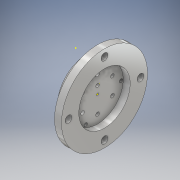
# Autodesk Inventor part: InnerSleeveFront
Saved by Autodesk Inventor 2017.3 (Build 213256000, 256)
## iProperties
Created: 2017-02-02
Part Number: InnerSleeveFront
Material: Generic
Document SubType Name: Modeling
Designer: Mac
Density: 1 g/cm^3
Appearance: Aluminum - Dark
Author: Mac
Autodesk Inventor part; units mm, degrees
ref_plane "YZ Plane" through (0, 0, 0) normal (1, 0, 0) x (0, 1, 0)
ref_plane "XZ Plane" through (0, 0, 0) normal (0, 1, 0) x (-1, 0, 0)
sketch "Sketch1" plane through (0, 0, 0) normal (1, 0, 0) x (0, 1, 0)
  circle A0 centre (0, 0) radius 13.2
  dimension "d0" = 26.4
  constraints: 1 centre point, 1 coincident
  measures "d0" diameter of A0
extrude "Extrusion1" add sketch "Sketch1" along normal blind 100
sketch "Sketch5" plane through (100, 0, 0) normal (1, 0, 0) x (0, 0, -1)
  line L0 (-14, -7) -> (14, -7)
  line L1 (14, -7) -> (14, 7)
  line L2 (14, 7) -> (-14, 7)
  line L3 (-14, 7) -> (-14, -7)
  line L4 (-7, -14) -> (7, -14)
  line L5 (7, -14) -> (7, 14)
  line L6 (7, 14) -> (-7, 14)
  line L7 (-7, 14) -> (-7, -14)
  point P0 (0, 0)
  constraints: 16 end point, 4 parallel, 2 horizontal, 2 perpendicular
move or copy body "Move Body1" bodies to move or copy 1 copy no translate (-5, 0, 0)
move or copy body "Move Body2" bodies to move or copy 1 copy no translate (10, 0, 0)
sketch "Sketch6" plane through (5, 0, 0) normal (-1, 0, 0) x (0, 0, 1)
  circle A0 centre (0, 0) radius 0.5
  dimension "d21" = 1
  constraints: 1 centre point, 1 coincident
  measures "d21" diameter of A0
extrude "Extrusion4" cut sketch "Sketch6" against normal blind 5
sketch "Sketch8" plane through (105, 0, 0) normal (1, 0, 0) x (0, 0, -1)
  circle A0 centre (0, 0) radius 11
  dimension "d35" = 22
  constraints: 1 centre point, 1 coincident
  measures "d35" diameter of A0
extrude "Extrusion6" cut sketch "Sketch8" against normal blind 95
extrude "Extrusion7" cut sketch "Sketch5" against normal blind 90
ref_plane "Work Plane4" through (5, 0, 13.2) normal (0, 0, 1) x (1, 0, 0)
ref_plane "Work Plane5" through (0, 0, -13.2) normal (0, 0, 1) x (1, 0, 0)
ref_plane "Work Plane11" through (5, 0, 0) normal (-1, 0, 0) x (0, 0, 1)
sketch "Sketch25" plane through (10, 0, 0) normal (1, 0, 0) x (0, 0, -1)
  circle A0 centre (-7.81, 0) radius 0.8 projected
  circle A1 centre (-7.81, 0) radius 0.8
  circle A2 centre (-3.905, -6.764) radius 0.835
  circle A3 centre (3.905, -6.764) radius 0.835
  circle A4 centre (7.81, 0) radius 0.835
  circle A5 centre (3.905, 6.764) radius 0.835
  circle A6 centre (-3.905, 6.7637) radius 0.8 projected
  circle A7 centre (-3.905, 6.7637) radius 0.835
  point P0 (0, 0)
  dimension "d96" = 1.67
  dimension "d97" = 1.67
  dimension "d98" = 1.67
  dimension "d99" = 1.67
  dimension "d100" = 1.67
  constraints: 6 centre point, 2 coincident
  measures "d96" diameter of A2
  measures "d97" diameter of A3
  measures "d98" diameter of A4
  measures "d99" diameter of A5
  measures "d100" diameter of A7
extrude "Extrusion8" cut sketch "Sketch25" against normal blind 4 contours A0 | A2 | A3 | A4 | A5 | A6
sketch "Sketch26" plane through (105, 0, 0) normal (1, 0, 0) x (0, 0, -1)
  point P0 (0, 0)
  point P1 (8.556, 8.556)
  point P2 (8.556, -8.556)
  point P3 (-8.556, -8.556)
  point P4 (-8.556, 8.556)
hole "Hole8" at (105, 8.556, -8.556) at (105, -8.556, -8.556) at (105, -8.556, 8.556) at (105, 8.556, 8.556) direction (-1, 0, 0) diameter 1.221 depth 2 tip angle 118 thread size "M1.6x0.35" class "6H" standard "ISO Metric profile"
ref_plane "Work Plane27" through (10, 0, 7.81) normal (0, -0.8660145, -0.5000189) x (-1, 0, 0)
ref_plane "Work Plane28" through (10, 6.7637, 3.905) normal (0, -0.8660241, 0.5000023) x (-1, 0, 0)
ref_plane "Work Plane29" through (10, -6.764, 3.905) normal (0, -0.8660145, -0.5000189) x (-1, 0, 0)
ref_plane "Work Plane30" through (10, 0, 7.81) normal (0, -0.8660145, 0.5000189) x (-1, 0, 0)
ref_plane "Work Plane31" through (10, 8.0496, 12.4577) normal (0, 0.8660145, 0.5000189) x (-1, 0, 0)
ref_plane "Work Plane32" through (10, -14.8136, -0.7427) normal (0, -0.8660145, -0.5000189) x (-1, 0, 0)
ref_plane "Work Plane33" through (10, 14.8134, -0.7425) normal (0, 0.8660241, -0.5000023) x (-1, 0, 0)
ref_plane "Work Plane34" through (10, -8.0496, 12.4577) normal (0, -0.8660145, 0.5000189) x (-1, 0, 0)
sketch "Sketch27" plane through (10, 14.8134, -0.7425) normal (0, 0.8660241, -0.5000023) x (-1, 0, 0)
  point P0 (10, -6.7637)
sketch "Sketch28" plane through (10, 14.8134, -0.7425) normal (0, 0.8660241, -0.5000023) x (-1, 0, 0)
  point P0 (10, -6.7637)
  point P1 (2, -6.764)
sketch "Sketch29" plane through (10, 8.0496, 12.4577) normal (0, 0.8660145, 0.5000189) x (-1, 0, 0)
  point P0 (10, -6.7636)
  point P1 (2, -6.764)
ref_plane "Work Plane35" through (10, 6.7637, 3.905) normal (0, 0, 1) x (-1, 0, 0)
ref_plane "Work Plane36" through (10, 6.764, -3.905) normal (0, 0, 1) x (-1, 0, 0)
ref_plane "Work Plane37" through (10, 6.7637, 13.2) normal (0, 0, 1) x (-1, 0, 0)
ref_plane "Work Plane38" through (10, 6.764, -13.2) normal (0, 0, -1) x (-1, 0, 0)
sketch "Sketch30" plane through (10, 6.7637, 13.2) normal (0, 0, 1) x (-1, 0, 0)
  point P0 (10, 6.7637)
sketch "Sketch31" plane through (10, -8.0496, 12.4577) normal (0, -0.8660145, 0.5000189) x (-1, 0, 0)
  point P0 (10, 6.7636)
  point P1 (2, 6.764)
sketch "Sketch32" plane through (10, -14.8136, -0.7427) normal (0, -0.8660145, -0.5000189) x (-1, 0, 0)
  point P0 (10, 6.7639)
  point P1 (2, 6.764)
sketch "Sketch33" plane through (10, 6.764, -13.2) normal (0, 0, -1) x (-1, 0, 0)
  point P0 (10, -6.764)
  point P1 (2, -6.764)
hole "Hole9" at (8, 11.4314, -6.6003) direction (0, -0.8660241, 0.5000023) diameter 1.221 depth 5.39 tip angle 118 thread size "M1.6x0.35" class "6H" standard "ISO Metric profile"
hole "Hole10" at (8, 11.4317, 6.6) direction (0, -0.8660145, -0.5000189) diameter 1.221 depth 5.39 tip angle 118 thread size "M1.6x0.35" class "6H" standard "ISO Metric profile"
hole "Hole12" at (8, -11.4317, 6.6) direction (0, 0.8660145, -0.5000189) diameter 1.221 depth 5.39 tip angle 118 thread size "M1.6x0.35" class "6H" standard "ISO Metric profile"
hole "Hole13" at (8, -11.4315, -6.6004) direction (0, 0.8660145, 0.5000189) diameter 1.221 depth 5.39 tip angle 118 thread size "M1.6x0.35" class "6H" standard "ISO Metric profile"
hole "Hole14" at (8, 0, -13.2) direction (0, 0, 1) diameter 1.221 depth 5.39 tip angle 118 thread size "M1.6x0.35" class "6H" standard "ISO Metric profile"
ref_plane "Work Plane42" through (10, 0, 0) normal (0, -0.7071222, 0.7070913) x (1, 0, 0)
ref_plane "Work Plane41" through (105, 9.3334, 9.3342) normal (0, 0.7070913, 0.7071222) x (-1, 0, 0)
ref_plane "Work Plane43" through (10, -9.334, 9.3336) normal (0, -0.7071222, 0.7070913) x (1, 0, 0)
ref_plane "Work Plane44" through (10, 9.334, -9.3336) normal (0, 0.7071222, -0.7070913) x (-1, 0, 0)
sketch "Sketch35" plane through (10, 9.334, -9.3336) normal (0, 0.7071222, -0.7070913) x (-1, 0, 0)
  point P0 (10, 0)
sketch "Sketch39" plane through (10, 0, 0) normal (1, 0, 0) x (0, 0, -1)
  point P0 (0, 0)
sketch "Sketch40" plane through (6, 0, 7.81) normal (1, 0, 0) x (0, 0, -1)
  circle A0 centre (0, 0) radius 0.8
  point P0 (7.81, 0)
  dimension "d192" = 1.6
  constraints: 1 centre point
  measures "d192" diameter of A0
extrude "Extrusion9" add sketch "Sketch40" along normal blind 4
sketch "Sketch44" plane through (5, 0, 0) normal (-1, 0, 0) x (0, 0, 1)
  point P0 (0, 0)
  point P1 (-15.3, -9.2926)
hole "Hole20" [suppressed]
sketch "Sketch45" plane through (10, 0, 0) normal (1, 0, 0) x (0, 0, -1)
  circle A0 centre (-3.5, 0) radius 0.8
  point P0 (0, 0)
  dimension "d213" = 1.6
  constraints: 1 centre point
  measures "d213" diameter of A0
extrude "Extrusion11" cut sketch "Sketch45" against normal blind 5
sketch "Sketch46" plane through (10, 0, 0) normal (1, 0, 0) x (0, 0, -1)
  point P0 (0, 0)
extrude "Extrusion12" [suppressed]
sketch "Sketch47" plane through (10, 0, 0) normal (1, 0, 0) x (0, 0, -1)
  circle A0 centre (-7.81, 0) radius 0.835
  point P0 (0, 0)
  dimension "d219" = 1.67
  constraints: 1 centre point
  measures "d219" diameter of A0
extrude "Extrusion13" cut sketch "Sketch47" against normal blind 4
sketch "Sketch48" plane through (105, 0, 0) normal (1, 0, 0) x (0, 0, -1)
  circle A0 centre (0, 0) radius 0.5 projected
  circle A1 centre (0, 0) radius 21.3351
  constraints: 1 centre point, 1 coincident
extrude "Extrusion14" cut sketch "Sketch48" against normal blind 95
sketch "Sketch49" plane through (10, 6.7637, 3.905) normal (0, 0, 1) x (-1, 0, 0)
  line L0 (0, 5.9287) -> (4, 5.9287) projected
  point P0 (10, 6.7637)
  point P1 (2, 5.9287)
  point P2 (2, 5.9287)
  constraints: 1 coincident, 1 midpoint
ref_plane "Work Plane46" through (10, 6.764, 13.2) normal (0, 0, 1) x (-1, 0, 0)
ref_plane "Work Plane45" through (10, 6.764, 13.345) normal (0, 0, 1) x (-1, 0, 0)
sketch "Sketch50" plane through (10, 6.764, 13.2) normal (0, 0, 1) x (-1, 0, 0)
  point P0 (10, 6.764)
sketch "Sketch51" plane through (10, 6.764, 13.2) normal (0, 0, 1) x (-1, 0, 0)
  point P0 (10, 6.764)
sketch "Sketch52" plane through (10, 6.764, 13.2) normal (0, 0, 1) x (-1, 0, 0)
  point P0 (10, 6.764)
  point P1 (2, 6.764)
hole "Hole21" at (8, 0, 13.2) direction (0, 0, -1) diameter 1.221 depth 5.3 tip angle 118 thread size "M1.6x0.35" class "6H" standard "ANSI Metric M Profile"
sketch "Sketch53" plane through (10, 0, 0) normal (1, 0, 0) x (0, 0, -1)
  circle A0 centre (0, 0) radius 0.5 projected
  circle A1 centre (0, 0) radius 11.7
  circle A2 centre (0, 0) radius 19.55
  dimension "d233" = 23.4
  dimension "d234" = 39.1
  constraints: 2 centre point, 2 coincident
  measures "d233" diameter of A1
  measures "d234" diameter of A2
extrude "Extrusion15" add sketch "Sketch53" along normal blind 3.175 contours A2
sketch "Sketch54" plane through (13.175, 0, 0) normal (1, 0, 0) x (0, 0, -1)
  circle A0 centre (-16.375, 0) radius 1.5875
  circle A1 centre (0, 16.375) radius 1.5875
  circle A2 centre (16.375, 0) radius 1.5875
  circle A3 centre (0, -16.375) radius 1.5875
  point P0 (0, 0)
  dimension "d237" = 3.175
  dimension "d238" = 3.175
  dimension "d239" = 3.175
  dimension "d240" = 3.175
  constraints: 4 centre point
  measures "d237" diameter of A0
  measures "d238" diameter of A1
  measures "d239" diameter of A2
  measures "d240" diameter of A3
extrude "Extrusion16" cut sketch "Sketch54" against normal blind 3.175
sketch "Sketch55" plane through (5, 0, 0) normal (-1, 0, 0) x (0, 0, 1)
  point P0 (0, 0)
  point P1 (0, 10.7)
  point P2 (9.266, -5.35)
  point P3 (-9.266, -5.35)
hole "Hole22" at (5, 10.7, 0) at (5, -5.35, -9.266) at (5, -5.35, 9.266) direction (1, 0, 0) diameter 1.567 depth 6.3 tip angle 118 thread size "M2x0.4" class "6H" standard "ISO Metric profile"
ref_plane "Work Plane39" through (105, -8.556, -8.556) normal (0, -0.7070913, -0.7071222) x (-1, 0, 0)
ref_plane "Work Plane40" through (105, -9.3338, -9.3338) normal (0, -0.7070913, -0.7071222) x (-1, 0, 0)
body "Solid1"
